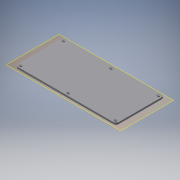
# Autodesk Inventor part: bottom
Saved by Autodesk Inventor 2017.3 (Build 213257000, 257)
## iProperties
Created: 2021-12-05
Part Number: bottom
Material: Generic
Document SubType Name: Modeling
Designer: TEOS
Density: 1 g/cm^3
Appearance: Default
Author: TEOS
Autodesk Inventor part; units mm, degrees
ref_plane "YZ Plane" through (0, 0, 0) normal (1, 0, 0) x (0, 1, 0)
ref_plane "XZ Plane" through (0, 0, 0) normal (0, 1, 0) x (-1, 0, 0)
ref_plane "XY Plane" through (0, 0, 0) normal (0, 0, 1) x (1, 0, 0)
ref_plane "Work Plane1" through (0, 0, -3) normal (0, 0, 1) x (1, 0, 0)
sketch "Sketch2" plane through (0, 0, -3) normal (0, 0, 1) x (1, 0, 0)
  circle A0 centre (-82, -37) radius 1 projected
  circle A1 centre (0, -37) radius 1 projected
  circle A2 centre (82, 37) radius 1 projected
  circle A3 centre (0, 37) radius 1 projected
  circle A4 centre (82, -37) radius 1 projected
  circle A5 centre (-82, 37) radius 1 projected
  arc A6 (-77, -37) -> (-82, -32) centre (-82, -37) ccw projected
  line L0 (-82, -32) -> (-82, 32) projected
  arc A7 (-82, 32) -> (-77, 37) centre (-82, 37) ccw projected
  line L1 (-77, 37) -> (-5, 37) projected
  arc A8 (-5, 37) -> (5, 37) centre (0, 37) ccw projected
  line L2 (5, 37) -> (77, 37) projected
  arc A9 (77, 37) -> (82, 32) centre (82, 37) ccw projected
  line L3 (82, 32) -> (82, -32) projected
  arc A10 (82, -32) -> (77, -37) centre (82, -37) ccw projected
  line L4 (77, -37) -> (5, -37) projected
  arc A11 (5, -37) -> (-5, -37) centre (0, -37) ccw projected
  line L5 (-5, -37) -> (-77, -37) projected
  line L6 (82, -42) -> (-82, -42) projected
  arc A12 (82, -42) -> (87, -37) centre (82, -37) ccw projected
  line L7 (87, 37) -> (87, -37) projected
  arc A13 (87, 37) -> (82, 42) centre (82, 37) ccw projected
  line L8 (-82, 42) -> (82, 42) projected
  arc A14 (-82, 42) -> (-87, 37) centre (-82, 37) ccw projected
  line L9 (-87, -37) -> (-87, 37) projected
  arc A15 (-87, -37) -> (-82, -42) centre (-82, -37) ccw projected
  point P0 (0, 0)
extrude "Extrusion1" add sketch "Sketch2" along normal blind 3 contours A6 L0 A7 L1 A8 L2 A9 L3 A10 L4 A11 L5 | L6 A15 L9 A14 L8 A13 L7 A12
sketch "Sketch3" plane through (0, 0, 0) normal (0, 0, 1) x (1, 0, 0)
  circle A0 centre (-82, 37) radius 1 projected
  circle A1 centre (82, -37) radius 1 projected
  circle A2 centre (0, 37) radius 1 projected
  circle A3 centre (82, 37) radius 1 projected
  circle A4 centre (0, -37) radius 1 projected
  circle A5 centre (-82, -37) radius 1 projected
  line L0 (-82, -42) -> (82, -42) projected
  arc A6 (82, -42) -> (87, -37) centre (82, -37) ccw projected
  line L1 (87, -37) -> (87, 37) projected
  arc A7 (87, 37) -> (82, 42) centre (82, 37) ccw projected
  line L2 (82, 42) -> (-82, 42) projected
  arc A8 (-82, 42) -> (-87, 37) centre (-82, 37) ccw projected
  line L3 (-87, 37) -> (-87, -37) projected
  arc A9 (-87, -37) -> (-82, -42) centre (-82, -37) ccw projected
  circle A10 centre (-82, 37) radius 1 projected
  circle A11 centre (82, 37) radius 1 projected
  point P0 (0, 0)
  constraints: 6 coincident
hole "Hole1" at (82, -37, 0) at (0, -37, 0) at (-82, -37, 0) at (-82, 37, 0) at (0, 37, 0) at (82, 37, 0) direction (0, 0, -1) diameter 3 depth 15 tip angle 118 countersink diameter 6 countersink angle 90
sketch "Sketch9" plane through (0, 0, -3) normal (0, 0, -1) x (-1, 0, 0)
  circle A0 centre (-28.4857, -17.7776) radius 1.5 projected
  circle A1 centre (-75.4853, -20.7832) radius 1.5 projected
  circle A2 centre (-62.2844, 31.2184) radius 1.5 projected
  circle A3 centre (-30.6986, 31.2222) radius 1.5 projected
  circle A4 centre (-28.4857, -17.7776) radius 3
  circle A5 centre (-75.4853, -20.7832) radius 3
  circle A6 centre (-30.6986, 31.2222) radius 3
  circle A7 centre (-62.2844, 31.2184) radius 3
  point P0 (0, 0)
  dimension "d38" = 6
  dimension "d39" = 6
  dimension "d40" = 6
  dimension "d41" = 6
  constraints: 4 centre point, 4 coincident
  measures "d38" diameter of A4
  measures "d39" diameter of A5
  measures "d40" diameter of A6
  measures "d41" diameter of A7
extrude "Extrusion4" add sketch "Sketch9" along normal blind 5 contours A0 | A1 | A2 | A3 | A4 | A5 | A6 | A7
sketch "Sketch10" plane through (28.4857, -17.7776, -8) normal (0, 0, -1) x (-1, 0, 0)
  circle A0 centre (0, 0) radius 3 projected
  circle A1 centre (-46.9996, -3.0056) radius 3 projected
  circle A2 centre (-33.7987, 48.996) radius 3 projected
  circle A3 centre (-2.2129, 48.9997) radius 3 projected
  point P0 (28.4857, 17.7776)
  point P1 (-2.2129, 48.9997)
  constraints: 4 coincident
hole "Hole2" at (28.4857, -17.7776, -8) at (30.6986, 31.2222, -8) at (62.2844, 31.2184, -8) at (75.4853, -20.7832, -8) direction (0, 0, 1) diameter 2 depth 5
ref_plane "Work Plane2" through (-56.5, 19.5, -27) normal (0, 0, 1) x (1, 0, 0)
sketch "Sketch11" plane through (-56.5, 19.5, -27) normal (0, 0, 1) x (1, 0, 0)
  circle A0 centre (-13.7, 0) radius 2.5 projected
  circle A1 centre (13.7, 0) radius 2.5 projected
  line L0 (25.7, -17.7) -> (25.7, 17.7) projected
  line L1 (25.7, 17.7) -> (-25.7, 17.7) projected
  line L2 (-25.7, 17.7) -> (-25.7, -17.7) projected
  line L3 (-25.7, -17.7) -> (25.7, -17.7) projected
  circle A2 centre (40.3, 0) radius 2.5 projected
  circle A3 centre (61.7, 0) radius 2.5 projected
  arc A4 (79.7, 4.408) -> (68.0785, -17.7) centre (105, -23) ccw projected
  line L4 (79.7, 4.408) -> (79.7, 17.7) projected
  line L5 (79.7, 17.7) -> (28.3, 17.7) projected
  line L6 (28.3, 17.7) -> (28.3, -17.7) projected
  line L7 (28.3, -17.7) -> (68.0785, -17.7) projected
  circle A5 centre (61.7, 0) radius 6
  circle A6 centre (40.3, 0) radius 6
  circle A7 centre (13.7, 0) radius 6
  circle A8 centre (-13.7, 0) radius 6
  line L8 (-25.7, 8) -> (79.7, 8)
  line L9 (79.7, 8) -> (79.7, -8)
  line L10 (79.7, -8) -> (-25.7, -8)
  line L11 (-25.7, -8) -> (-25.7, 8)
  point P0 (56.5, -19.5)
  dimension "d51" = 12
  dimension "d52" = 12
  dimension "d53" = 12
  dimension "d54" = 12
  dimension "d55" = 16
  dimension "d56" = 105.4
  dimension "d57" = 8
  constraints: 8 end point, 4 centre point, 4 coincident, 2 parallel, 1 horizontal, 1 perpendicular, 1 point on line
  measures "d51" diameter of A5
  measures "d52" diameter of A6
  measures "d53" diameter of A7
  measures "d54" diameter of A8
  measures "d55" distance between parallel lines of L10 L8
  measures "d56" distance of L8.start L8.end
  measures "d57" distance from line of A0.centre L8
extrude "Extrusion5" add sketch "Sketch11" along normal blind 3 contours L10 L2 L8 L0 | L0 L8 L6 L10 | L6 L8 L4 A4 L10 | A4 L9 L10
sketch "Sketch12" plane through (23.2, 11.5, -27) normal (1, 0, 0) x (0, 0, -1)
  line L0 (-3, 0) -> (-3, 16) projected
  line L1 (-24, 25.5) -> (-24, -48.5) projected
  line L2 (-3, 16) -> (-24, 16)
  line L3 (-24, -48.5) -> (-24, 25.5) projected
  line L4 (-3, 0) -> (-24, 0)
  line L5 (-24, 0) -> (-24, 16)
  line L6 (-3, 16) -> (-3, 0)
  point P0 (-27, -11.5)
  constraints: 8 end point, 2 collinear, 2 perpendicular, 2 point on line
extrude "Extrusion6" add sketch "Sketch12" against normal blind 3
sketch "Sketch13" plane through (-82.2, 11.5, -27) normal (-1, 0, 0) x (0, 0, 1)
  line L0 (3, 0) -> (3, 16) projected
  line L1 (3, 0) -> (24, 0) projected
  line L2 (24, 16) -> (24, 0) projected
  line L3 (24, 16) -> (3, 16) projected
  point P0 (27, -11.5)
extrude "Extrusion7" add sketch "Sketch13" against normal blind 3
ref_plane "Work Plane3" through (-29.5, 11.5, -27) normal (1, 0, 0) x (0, 0, -1)
sketch "Sketch14" plane through (-29.5, 11.5, -27) normal (1, 0, 0) x (0, 0, -1)
  line L0 (-3, 16) -> (-3, 0) projected
  line L1 (-3, 16) -> (-24, 16) projected
  line L2 (-24, 0) -> (-24, 16) projected
  line L3 (-24, 0) -> (-3, 0) projected
  point P0 (-27, -11.5)
extrude "Extrusion8" add sketch "Sketch14" along normal blind 1.5 and the other way blind 1.5
equation "\"d26\" = 55deg"
equation "\"Sketch6_Pitch\" = 3"
body "Solid1"
